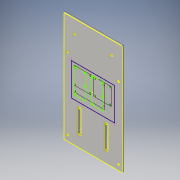
# Autodesk Inventor part: Part2
Saved by Autodesk Inventor 2016 (Build 200138000, 138)
## iProperties
Created: 2015-10-15
Part Number: Part2
Material: Generic
Document SubType Name: Modeling
Designer: hozhu
Density: 1 g/cm^3
Appearance: Default
Author: hozhu
Autodesk Inventor part; units mm, degrees
ref_plane "YZ Plane" through (0, 0, 0) normal (1, 0, 0) x (0, 1, 0)
ref_plane "XZ Plane" through (0, 0, 0) normal (0, 1, 0) x (-1, 0, 0)
ref_plane "XY Plane" through (0, 0, 0) normal (0, 0, 1) x (1, 0, 0)
sketch "Sketch1" plane through (0, 0, 0) normal (0, 0, 1) x (1, 0, 0)
  line L0 (-68.58, -128.7145) -> (68.58, -128.7145)
  line L1 (68.58, -128.7145) -> (68.58, 128.7145)
  line L2 (68.58, 128.7145) -> (-68.58, 128.7145)
  line L3 (-68.58, 128.7145) -> (-68.58, -128.7145)
  line L4 (-68.58, -128.7145) -> (68.58, 128.7145) construction
  line L5 (68.58, -128.7145) -> (-68.58, 128.7145) construction
  point P0 (0, 0)
  dimension "d0" = 137.16
  dimension "d1" = 257.429
  constraints: 12 end point, 2 midpoint, 2 parallel, 1 horizontal, 1 perpendicular
  measures "d0" distance of L1.end L2.end
  measures "d1" distance of L2.end L0.start
extrude "Extrusion1" add sketch "Sketch1" against normal blind 3.175
sketch "Sketch2" plane through (0, 0, 0) normal (0, 0, 1) x (1, 0, 0)
  circle A0 centre (-59.69, 52.5145) radius 2.0955
  line L0 (-68.58, 128.7145) -> (-68.58, -128.7145) projected
  line L1 (-68.58, 128.7145) -> (68.58, 128.7145) projected
  circle A1 centre (59.69, 52.5145) radius 2.0955
  line L2 (68.58, -128.7145) -> (68.58, 128.7145) projected
  circle A2 centre (-59.69, -116.0145) radius 2.0955
  circle A3 centre (59.69, -116.0145) radius 2.0955
  line L3 (-68.58, -128.7145) -> (68.58, -128.7145) projected
  point P0 (0, 0)
  dimension "d4" = 8.89
  dimension "d5" = 76.2
  dimension "d6" = 76.2
  dimension "d7" = 8.89
  dimension "d8" = 4.191
  dimension "d9" = 12.7
  dimension "d10" = 8.89
  dimension "d11" = 8.89
  dimension "d12" = 12.7
  dimension "d13" = 4.191
  dimension "d21" = 4.191
  dimension "d22" = 4.191
  constraints: 4 centre point
  measures "d4" distance from line of L0 A0.centre
  measures "d5" distance from line of L1 A0.centre
  measures "d6" distance from line of L1 A1.centre
  measures "d7" distance from line of A1.centre L2
  measures "d8" diameter of A1
  measures "d9" distance from line of L3 A2.centre
  measures "d10" distance from line of L0 A2.centre
  measures "d11" distance from line of L2 A3.centre
  measures "d12" distance from line of L3 A3.centre
  measures "d13" diameter of A0
  measures "d21" diameter of A2
  measures "d22" diameter of A3
hole "Hole1" at (-59.69, 52.5145, 0) at (59.69, 52.5145, 0) at (-59.69, -116.0145, 0) at (59.69, -116.0145, 0) direction (0, 0, -1) diameter 4.191 end through all
sketch "Sketch4" plane through (0, 0, 0) normal (0, 0, 1) x (1, 0, 0)
  line L0 (-35.179, -49.0855) -> (-35.179, -99.8855)
  line L1 (-28.321, -49.0855) -> (-28.321, -99.8855)
  line L2 (28.321, -49.0855) -> (28.321, -99.8855)
  line L3 (35.179, -49.0855) -> (35.179, -99.8855)
  line L4 (-68.58, 128.7145) -> (-68.58, -128.7145) projected
  line L5 (68.58, -128.7145) -> (68.58, 128.7145) projected
  line L6 (-68.58, -128.7145) -> (68.58, -128.7145) projected
  arc A0 (-28.321, -49.0855) -> (-35.179, -49.0855) centre (-31.75, -49.0855) ccw
  arc A1 (-35.179, -99.8855) -> (-28.321, -99.8855) centre (-31.75, -99.8855) ccw
  arc A2 (35.179, -49.0855) -> (28.321, -49.0855) centre (31.75, -49.0855) ccw
  arc A3 (28.321, -99.8855) -> (35.179, -99.8855) centre (31.75, -99.8855) ccw
  point P0 (0, 0)
  dimension "d23" = 6.858
  dimension "d24" = 6.858
  dimension "d25" = 33.401
  dimension "d26" = 50.8
  dimension "d27" = 33.401
  dimension "d28" = 28.829
  dimension "d29" = 28.829
  dimension "d30" = 28.829
  dimension "d31" = 28.829
  dimension "d32" = 50.8
  dimension "d33" = 50.8
  dimension "d34" = 50.8
  constraints: 8 end point, 8 point on circle, 4 centre point, 4 tangent, 4 vertical
  measures "d23" distance of L1.end L0.end
  measures "d24" distance between parallel lines of L3 L2
  measures "d25" distance between parallel lines of L4 L0
  measures "d26" distance of L3.start L3.end
  measures "d27" distance between parallel lines of L5 L3
  measures "d28" distance from line of L6 L0.end
  measures "d29" distance from line of L6 L1.end
  measures "d30" distance from line of L6 L2.end
  measures "d31" distance from line of L6 L3.end
  measures "d32" distance of L0.start L0.end
  measures "d33" distance of L1.start L1.end
  measures "d34" distance of L2.start L2.end
extrude "Extrusion2" cut sketch "Sketch4" against normal blind 3.175
sketch "Sketch5" plane through (0, 0, 0) normal (0, 0, 1) x (1, 0, 0)
  line L0 (-68.58, 128.7145) -> (68.58, 128.7145) projected
  line L1 (68.58, 128.7145) -> (68.58, -128.7145) projected
  point P0 (0, 0)
  point P1 (-43.3324, 96.9645)
  point P2 (43.3324, 96.9645)
  dimension "d37" = 31.75
  dimension "d38" = 86.6648
  dimension "d39" = 31.75
  dimension "d40" = 25.2476
  measures "d37" distance from line of L0 point (-43.332, 96.964)
  measures "d38" distance of point (-43.332, 96.964) point (43.332, 96.964)
  measures "d39" distance from line of L0 point (43.332, 96.964)
  measures "d40" distance from line of L1 point (43.332, 96.964)
hole "Hole2" at (-43.3324, 96.9645, 0) at (43.3324, 96.9645, 0) direction (0, 0, -1) diameter 4.4704 end through all
sketch "smartsensorPowered" plane through (0, 0, 0) normal (0, 0, 1) x (1, 0, 0)
  line L0 (-68.58, 128.7145) -> (-68.58, -128.7145) projected
  line L1 (68.58, 128.7145) -> (-68.58, 128.7145) projected
  line L2 (68.58, -128.7145) -> (68.58, 128.7145) projected
  line L3 (-44.45, 33.4645) -> (-16.51, 33.4645)
  line L4 (-16.51, 33.4645) -> (-16.51, -26.2255)
  line L5 (-16.51, -26.2255) -> (-44.45, -26.2255)
  line L6 (-44.45, -26.2255) -> (-44.45, 33.4645)
  circle A0 centre (-41.275, 30.2895) radius 1.651
  circle A1 centre (-40.64, -22.4155) radius 1.651
  circle A2 centre (-19.685, 2.9845) radius 1.651
  circle A3 centre (-19.685, 30.2895) radius 1.651
  line L7 (-3.81, 33.4645) -> (24.13, 33.4645)
  line L8 (24.13, 33.4645) -> (24.13, -26.2255)
  line L9 (24.13, -26.2255) -> (-3.81, -26.2255)
  line L10 (-3.81, -26.2255) -> (-3.81, 33.4645)
  circle A4 centre (-0.635, 30.2895) radius 1.651
  circle A5 centre (0, -22.4155) radius 1.651
  circle A6 centre (20.955, 2.9845) radius 1.651
  circle A7 centre (20.955, 30.2895) radius 1.651
  point P0 (0, 0)
  dimension "d52" = 27.94
  dimension "d53" = 59.69
  dimension "d59" = 3.175
  dimension "d60" = 3.175
  dimension "d61" = 3.302
  dimension "d62" = 3.302
  dimension "d63" = 3.175
  dimension "d64" = 3.175
  dimension "d66" = 3.81
  dimension "d67" = 3.81
  dimension "d68" = 3.302
  dimension "d69" = 30.48
  dimension "d70" = 3.175
  dimension "d71" = 3.302
  dimension "d72" = 27.94
  dimension "d73" = 59.69
  dimension "d74" = 3.175
  dimension "d75" = 3.175
  dimension "d76" = 3.302
  dimension "d77" = 3.302
  dimension "d78" = 3.175
  dimension "d79" = 3.175
  dimension "d80" = 3.81
  dimension "d81" = 3.81
  dimension "d82" = 3.302
  dimension "d83" = 30.48
  dimension "d84" = 3.175
  dimension "d85" = 3.302
  dimension "d86" = 12.7
  constraints: 16 end point, 8 centre point, 4 parallel, 2 horizontal, 2 perpendicular, 1 collinear
  measures "d52" distance of L3.start L3.end
  measures "d53" distance of L5.end L3.start
  measures "d59" distance from line of L6 A0.centre
  measures "d60" distance from line of A0.centre L3
  measures "d61" diameter of A0
  measures "d62" diameter of A3
  measures "d63" distance from line of L4 A3.centre
  measures "d64" distance from line of L3 A3.centre
  measures "d66" distance from line of L5 A1.centre
  measures "d67" distance from line of L6 A1.centre
  measures "d68" diameter of A1
  measures "d69" distance from line of L3 A2.centre
  measures "d70" distance from line of L4 A2.centre
  measures "d71" diameter of A2
  measures "d72" distance of L10.end L7.end
  measures "d73" distance of L10.start L10.end
  measures "d74" distance from line of L10 A4.centre
  measures "d75" distance from line of A4.centre L7
  measures "d76" diameter of A4
  measures "d77" diameter of A7
  measures "d78" distance from line of L8 A7.centre
  measures "d79" distance from line of L7 A7.centre
  measures "d80" distance from line of L9 A5.centre
  measures "d81" distance from line of L10 A5.centre
  measures "d82" diameter of A5
  measures "d83" distance from line of L7 A6.centre
  measures "d84" distance from line of L8 A6.centre
  measures "d85" diameter of A6
  measures "d86" distance between parallel lines of L10 L4
sketch "BoardArea" plane through (0, 0, 0) normal (0, 0, 1) x (1, 0, 0)
  line L0 (-50.8, 39.8145) -> (50.8, 39.8145)
  line L1 (50.8, 39.8145) -> (50.8, -36.3855)
  line L2 (50.8, -36.3855) -> (-50.8, -36.3855)
  line L3 (-50.8, -36.3855) -> (-50.8, 39.8145)
  point P0 (0, 0)
  constraints: 8 end point, 2 parallel, 1 horizontal, 1 perpendicular
sketch "teamflag" plane through (0, 0, 0) normal (0, 0, 1) x (1, 0, 0)
  line L0 (-3.81, -7.1755) -> (-44.45, -7.1755)
  line L1 (-44.45, -7.1755) -> (-44.45, 33.4645)
  line L2 (-44.45, 33.4645) -> (-3.81, 33.4645)
  line L3 (-3.81, 33.4645) -> (-3.81, -7.1755)
  circle A0 centre (-6.35, 30.9245) radius 1.651
  circle A1 centre (-41.91, 30.9245) radius 1.651
  circle A2 centre (-41.91, -4.6355) radius 1.651
  circle A3 centre (-6.35, -4.6355) radius 1.651
  line L4 (-50.8, -36.3855) -> (-50.8, 39.8145) projected
  circle A4 centre (-43.3324, 96.9645) radius 2.2352 projected
  circle A5 centre (43.3324, 96.9645) radius 2.2352 projected
  arc A6 (-35.179, -99.8855) -> (-28.321, -99.8855) centre (-31.75, -99.8855) ccw projected
  line L5 (-28.321, -99.8855) -> (-28.321, -49.0855) projected
  arc A7 (-28.321, -49.0855) -> (-35.179, -49.0855) centre (-31.75, -49.0855) ccw projected
  line L6 (-35.179, -49.0855) -> (-35.179, -99.8855) projected
  arc A8 (28.321, -99.8855) -> (35.179, -99.8855) centre (31.75, -99.8855) ccw projected
  line L7 (35.179, -99.8855) -> (35.179, -49.0855) projected
  arc A9 (35.179, -49.0855) -> (28.321, -49.0855) centre (31.75, -49.0855) ccw projected
  line L8 (28.321, -49.0855) -> (28.321, -99.8855) projected
  circle A10 centre (-59.69, -116.0145) radius 2.0955 projected
  circle A11 centre (-59.69, 52.5145) radius 2.0955 projected
  circle A12 centre (59.69, 52.5145) radius 2.0955 projected
  circle A13 centre (59.69, -116.0145) radius 2.0955 projected
  line L9 (68.58, 128.7145) -> (68.58, -128.7145) projected
  line L10 (68.58, -128.7145) -> (-68.58, -128.7145) projected
  line L11 (-68.58, -128.7145) -> (-68.58, 128.7145) projected
  line L12 (-68.58, 128.7145) -> (68.58, 128.7145) projected
  circle A14 centre (-43.3324, 96.9645) radius 2.2352 projected
  circle A15 centre (43.3324, 96.9645) radius 2.2352 projected
  arc A16 (-35.179, -99.8855) -> (-28.321, -99.8855) centre (-31.75, -99.8855) ccw projected
  line L13 (-28.321, -99.8855) -> (-28.321, -49.0855) projected
  arc A17 (-28.321, -49.0855) -> (-35.179, -49.0855) centre (-31.75, -49.0855) ccw projected
  line L14 (-35.179, -49.0855) -> (-35.179, -99.8855) projected
  arc A18 (28.321, -99.8855) -> (35.179, -99.8855) centre (31.75, -99.8855) ccw projected
  line L15 (35.179, -99.8855) -> (35.179, -49.0855) projected
  arc A19 (35.179, -49.0855) -> (28.321, -49.0855) centre (31.75, -49.0855) ccw projected
  line L16 (28.321, -49.0855) -> (28.321, -99.8855) projected
  circle A20 centre (-59.69, -116.0145) radius 2.0955 projected
  circle A21 centre (-59.69, 52.5145) radius 2.0955 projected
  circle A22 centre (59.69, 52.5145) radius 2.0955 projected
  circle A23 centre (59.69, -116.0145) radius 2.0955 projected
  line L17 (68.58, 128.7145) -> (68.58, -128.7145) projected
  line L18 (68.58, -128.7145) -> (-68.58, -128.7145) projected
  line L19 (-68.58, -128.7145) -> (-68.58, 128.7145) projected
  line L20 (-68.58, 128.7145) -> (68.58, 128.7145) projected
  circle A24 centre (-43.3324, 96.9645) radius 2.2352 projected
  circle A25 centre (43.3324, 96.9645) radius 2.2352 projected
  arc A26 (-35.179, -99.8855) -> (-28.321, -99.8855) centre (-31.75, -99.8855) ccw projected
  line L21 (-28.321, -99.8855) -> (-28.321, -49.0855) projected
  arc A27 (-28.321, -49.0855) -> (-35.179, -49.0855) centre (-31.75, -49.0855) ccw projected
  line L22 (-35.179, -49.0855) -> (-35.179, -99.8855) projected
  arc A28 (28.321, -99.8855) -> (35.179, -99.8855) centre (31.75, -99.8855) ccw projected
  line L23 (35.179, -99.8855) -> (35.179, -49.0855) projected
  arc A29 (35.179, -49.0855) -> (28.321, -49.0855) centre (31.75, -49.0855) ccw projected
  line L24 (28.321, -49.0855) -> (28.321, -99.8855) projected
  circle A30 centre (-59.69, -116.0145) radius 2.0955 projected
  circle A31 centre (-59.69, 52.5145) radius 2.0955 projected
  circle A32 centre (59.69, 52.5145) radius 2.0955 projected
  circle A33 centre (59.69, -116.0145) radius 2.0955 projected
  line L25 (68.58, 128.7145) -> (68.58, -128.7145) projected
  line L26 (68.58, -128.7145) -> (-68.58, -128.7145) projected
  line L27 (-68.58, -128.7145) -> (-68.58, 128.7145) projected
  line L28 (-68.58, 128.7145) -> (68.58, 128.7145) projected
  circle A34 centre (-43.3324, 96.9645) radius 2.2352 projected
  circle A35 centre (43.3324, 96.9645) radius 2.2352 projected
  arc A36 (-35.179, -99.8855) -> (-28.321, -99.8855) centre (-31.75, -99.8855) ccw projected
  line L29 (-28.321, -99.8855) -> (-28.321, -49.0855) projected
  arc A37 (-28.321, -49.0855) -> (-35.179, -49.0855) centre (-31.75, -49.0855) ccw projected
  line L30 (-35.179, -49.0855) -> (-35.179, -99.8855) projected
  arc A38 (28.321, -99.8855) -> (35.179, -99.8855) centre (31.75, -99.8855) ccw projected
  line L31 (35.179, -99.8855) -> (35.179, -49.0855) projected
  arc A39 (35.179, -49.0855) -> (28.321, -49.0855) centre (31.75, -49.0855) ccw projected
  line L32 (28.321, -49.0855) -> (28.321, -99.8855) projected
  circle A40 centre (-59.69, -116.0145) radius 2.0955 projected
  circle A41 centre (-59.69, 52.5145) radius 2.0955 projected
  circle A42 centre (59.69, 52.5145) radius 2.0955 projected
  circle A43 centre (59.69, -116.0145) radius 2.0955 projected
  line L33 (68.58, 128.7145) -> (68.58, -128.7145) projected
  line L34 (68.58, -128.7145) -> (-68.58, -128.7145) projected
  line L35 (-68.58, -128.7145) -> (-68.58, 128.7145) projected
  line L36 (-68.58, 128.7145) -> (68.58, 128.7145) projected
  circle A44 centre (-43.3324, 96.9645) radius 2.2352 projected
  circle A45 centre (43.3324, 96.9645) radius 2.2352 projected
  arc A46 (-35.179, -99.8855) -> (-28.321, -99.8855) centre (-31.75, -99.8855) ccw projected
  line L37 (-28.321, -99.8855) -> (-28.321, -49.0855) projected
  arc A47 (-28.321, -49.0855) -> (-35.179, -49.0855) centre (-31.75, -49.0855) ccw projected
  line L38 (-35.179, -49.0855) -> (-35.179, -99.8855) projected
  arc A48 (28.321, -99.8855) -> (35.179, -99.8855) centre (31.75, -99.8855) ccw projected
  line L39 (35.179, -99.8855) -> (35.179, -49.0855) projected
  arc A49 (35.179, -49.0855) -> (28.321, -49.0855) centre (31.75, -49.0855) ccw projected
  line L40 (28.321, -49.0855) -> (28.321, -99.8855) projected
  circle A50 centre (-59.69, -116.0145) radius 2.0955 projected
  circle A51 centre (-59.69, 52.5145) radius 2.0955 projected
  circle A52 centre (59.69, 52.5145) radius 2.0955 projected
  circle A53 centre (59.69, -116.0145) radius 2.0955 projected
  line L41 (68.58, 128.7145) -> (68.58, -128.7145) projected
  line L42 (68.58, -128.7145) -> (-68.58, -128.7145) projected
  line L43 (-68.58, -128.7145) -> (-68.58, 128.7145) projected
  line L44 (-68.58, 128.7145) -> (68.58, 128.7145) projected
  line L45 (-50.8, 39.8145) -> (50.8, 39.8145) projected
  line L46 (43.18, -7.1755) -> (2.54, -7.1755)
  line L47 (2.54, -7.1755) -> (2.54, 33.4645)
  line L48 (2.54, 33.4645) -> (43.18, 33.4645)
  line L49 (43.18, 33.4645) -> (43.18, -7.1755)
  circle A54 centre (40.64, 30.9245) radius 1.651
  circle A55 centre (5.08, 30.9245) radius 1.651
  circle A56 centre (5.08, -4.6355) radius 1.651
  circle A57 centre (40.64, -4.6355) radius 1.651
  dimension "d100" = 3.302
  dimension "d101" = 40.64
  dimension "d102" = 40.64
  dimension "d103" = 2.54
  dimension "d104" = 2.54
  dimension "d105" = 2.54
  dimension "d106" = 38.1
  dimension "d107" = 38.1
  dimension "d108" = 2.54
  dimension "d109" = 38.1
  dimension "d110" = 38.1
  dimension "d113" = 3.302
  dimension "d114" = 40.64
  dimension "d115" = 40.64
  dimension "d116" = 2.54
  dimension "d117" = 2.54
  dimension "d118" = 2.54
  dimension "d119" = 38.1
  dimension "d120" = 38.1
  dimension "d121" = 2.54
  dimension "d122" = 38.1
  dimension "d123" = 38.1
  dimension "d124" = 6.35
  constraints: 16 end point, 8 centre point, 6 equal radius, 4 parallel, 2 horizontal, 2 vertical, 1 collinear
  measures "d100" diameter of A0
  measures "d101" distance between parallel lines of L1 L3
  measures "d102" distance between parallel lines of L2 L0
  measures "d103" distance from line of A0.centre L3
  measures "d104" distance from line of A0.centre L2
  measures "d105" distance from line of A3.centre L3
  measures "d106" distance from line of A3.centre L2
  measures "d107" distance from line of A1.centre L3
  measures "d108" distance from line of A1.centre L2
  measures "d109" distance from line of A2.centre L3
  measures "d110" distance from line of A2.centre L2
  measures "d113" diameter of A54
  measures "d114" distance between parallel lines of L47 L49
  measures "d115" distance between parallel lines of L48 L46
  measures "d116" distance from line of A54.centre L49
  measures "d117" distance from line of A54.centre L48
  measures "d118" distance from line of A57.centre L49
  measures "d119" distance from line of A57.centre L48
  measures "d120" distance from line of A55.centre L49
  measures "d121" distance from line of A55.centre L48
  measures "d122" distance from line of A56.centre L49
  measures "d123" distance from line of A56.centre L48
  measures "d124" distance between parallel lines of L47 L3
sketch "cape" plane through (0, 0, 0) normal (0, 0, 1) x (1, 0, 0)
  line L0 (-44.45, -21.1355) -> (27.61, -21.1355)
  line L1 (27.61, -21.1355) -> (27.61, 33.4645)
  line L2 (27.61, 33.4645) -> (-44.45, 33.4645)
  line L3 (-44.45, 33.4645) -> (-44.45, -21.1355)
  circle A0 centre (-41.275, -17.9605) radius 1.5875
  circle A1 centre (24.765, -14.7855) radius 1.5875
  circle A2 centre (24.765, 27.1245) radius 1.5875
  circle A3 centre (-41.275, 30.2995) radius 1.5875
  line L4 (-50.8, 39.8145) -> (50.8, 39.8145) projected
  line L5 (-50.8, -36.3855) -> (-50.8, 39.8145) projected
  point P0 (0, 0)
  dimension "d125" = 3.175
  dimension "d126" = 72.06
  dimension "d127" = 54.6
  dimension "d130" = 2.845
  dimension "d131" = 6.34
  dimension "d132" = 2.845
  dimension "d133" = 48.25
  dimension "d134" = 68.885
  dimension "d135" = 3.165
  dimension "d136" = 68.885
  dimension "d137" = 51.425
  constraints: 8 end point, 4 centre point, 3 equal radius, 2 parallel, 1 horizontal, 1 vertical
  measures "d125" diameter of A2
  measures "d126" distance between parallel lines of L1 L3
  measures "d127" distance between parallel lines of L2 L0
  measures "d130" distance from line of A2.centre L1
  measures "d131" distance from line of A2.centre L2
  measures "d132" distance from line of A1.centre L1
  measures "d133" distance from line of A1.centre L2
  measures "d134" distance from line of A3.centre L1
  measures "d135" distance from line of A3.centre L2
  measures "d136" distance from line of A0.centre L1
  measures "d137" distance from line of A0.centre L2
body "Solid1"
